Autodesk Fusion 360 part; units mm, degrees
note: some values were not read from the file. Chosen so that the rebuilt part matches the saved one: which bodies a step acts on; which face or edge a step refers to.
(part 2 of 3)
sketch "Sketch11 (2)" plane through (0, 171.45, 0) normal (0, 1, 0) x (-1, 0, 0) in component "enclosure"
  line L0 (75.40625, 30.353) -> (75.40625, -30.353)
  arc A0 (73.2155, -32.54375) -> (75.40625, -30.353) centre (73.2155, -30.353) ccw
  line L1 (73.2155, -32.54375) -> (-73.2155, -32.54375)
  arc A1 (-75.40625, -30.353) -> (-73.2155, -32.54375) centre (-73.2155, -30.353) ccw
  line L2 (-75.40625, -30.353) -> (-75.40625, 30.353)
  arc A2 (-73.2155, 32.54375) -> (-75.40625, 30.353) centre (-73.2155, 30.353) ccw
  line L3 (-73.2155, 32.54375) -> (73.2155, 32.54375)
  arc A3 (75.40625, 30.353) -> (73.2155, 32.54375) centre (73.2155, 30.353) ccw
  arc A4 (73.2155, -34.925) -> (77.7875, -30.353) centre (73.2155, -30.353) ccw
  line L4 (77.7875, -30.353) -> (77.7875, 30.353)
  arc A5 (77.7875, 30.353) -> (73.2155, 34.925) centre (73.2155, 30.353) ccw
  line L5 (73.2155, 34.925) -> (-73.2155, 34.925)
  arc A6 (-73.2155, 34.925) -> (-77.7875, 30.353) centre (-73.2155, 30.353) ccw
  line L6 (-77.7875, 30.353) -> (-77.7875, -30.353)
  arc A7 (-77.7875, -30.353) -> (-73.2155, -34.925) centre (-73.2155, -30.353) ccw
  line L7 (-73.2155, -34.925) -> (73.2155, -34.925)
  line L8 (-73.2155, 32.54375) -> (73.2155, 32.54375)
  line L9 (73.2155, 32.54375) -> (-73.2155, 32.54375)
  line L10 (73.2155, -32.54375) -> (-73.2155, -32.54375)
  line L11 (-73.2155, -32.54375) -> (73.2155, -32.54375)
  line L12 (-75.40625, -30.353) -> (-75.40625, 30.353)
  line L13 (-75.40625, 30.353) -> (-75.40625, -30.353)
  line L14 (75.40625, 30.353) -> (75.40625, -30.353)
  line L15 (75.40625, -30.353) -> (75.40625, 30.353)
  line L16 (0, 32.54375) -> (0, -32.54375) construction
  line L17 (-75.40625, 0) -> (0, 0) construction
  line L18 (-75.40625, 6.35) -> (-75.40625, -6.35)
  line L19 (-73.025, -3.96875) -> (-73.025, 3.96875)
  line L20 (-73.025, 6.35) -> (-75.40625, -6.35) construction
  line L21 (-75.40625, 6.35) -> (-73.025, -6.35) construction
  arc A8 (-73.025, 3.96875) -> (-75.40625, 6.35) centre (-75.40625, 3.96875) ccw
  arc A9 (-75.40625, -6.35) -> (-73.025, -3.96875) centre (-75.40625, -3.96875) ccw
  line L22 (73.025, -3.96875) -> (73.025, 3.96875)
  arc A10 (75.40625, 6.35) -> (73.025, 3.96875) centre (75.40625, 3.96875) ccw
  arc A11 (73.025, -3.96875) -> (75.40625, -6.35) centre (75.40625, -3.96875) ccw
  line L23 (75.40625, 6.35) -> (75.40625, -6.35)
  point P0 (-74.215625, 0)
  dimension "d154" = 12.7
  dimension "d155" = 2.38125
  dimension "d156" = 2.38125
  dimension "d157" = 2.38125
  constraint coincident L17.end origin
  constraint parallel L18 L19
  constraint coincident L20.start L19
  constraint tangent L19 A8
  constraint coincident L21.end L19
  constraint tangent L19 A9
  constraint collinear L2 L18
  constraint symmetric L16 A8 A10
  constraint symmetric L16 A9 A11
  measures "d156" radius of A8
  measures "d157" radius of A9
extrude "Extrude8'" add sketch "Sketch11 (2)" against normal up to surface (169.8625 mm away) contours L0 L14 L15 L22 A10 A11 L23 | L2 L12 L13 L18 L19 A8 A9 picked at (74.6125, -1.322917) picked at (-74.6125, -1.322917) bodies 2 in component "enclosure"
sketch "Sketch12" plane through (0, 171.45, 0) normal (0, 1, 0) x (-1, 0, 0) in component "enclosure"
  line L0 (75.40625, 30.353) -> (75.40625, 6.35)
  arc A0 (75.40625, 6.35) -> (73.025, 3.96875) centre (75.40625, 3.96875) ccw
  line L1 (73.025, 3.96875) -> (73.025, -3.96875)
  arc A1 (73.025, -3.96875) -> (75.40625, -6.35) centre (75.40625, -3.96875) ccw
  line L2 (75.40625, -6.35) -> (75.40625, -30.353)
  arc A2 (73.2155, -32.54375) -> (75.40625, -30.353) centre (73.2155, -30.353) ccw
  line L3 (73.2155, -32.54375) -> (-73.2155, -32.54375)
  arc A3 (-75.40625, -30.353) -> (-73.2155, -32.54375) centre (-73.2155, -30.353) ccw
  line L4 (-75.40625, -30.353) -> (-75.40625, -6.35)
  arc A4 (-75.40625, -6.35) -> (-73.025, -3.96875) centre (-75.40625, -3.96875) ccw
  line L5 (-73.025, -3.96875) -> (-73.025, 3.96875)
  arc A5 (-73.025, 3.96875) -> (-75.40625, 6.35) centre (-75.40625, 3.96875) ccw
  line L6 (-75.40625, 6.35) -> (-75.40625, 30.353)
  arc A6 (-73.2155, 32.54375) -> (-75.40625, 30.353) centre (-73.2155, 30.353) ccw
  line L7 (-73.2155, 32.54375) -> (73.2155, 32.54375)
  arc A7 (75.40625, 30.353) -> (73.2155, 32.54375) centre (73.2155, 30.353) ccw
  arc A8 (73.2155, -34.925) -> (77.7875, -30.353) centre (73.2155, -30.353) ccw
  line L8 (77.7875, -30.353) -> (77.7875, 30.353)
  arc A9 (77.7875, 30.353) -> (73.2155, 34.925) centre (73.2155, 30.353) ccw
  line L9 (73.2155, 34.925) -> (-73.2155, 34.925)
  arc A10 (-73.2155, 34.925) -> (-77.7875, 30.353) centre (-73.2155, 30.353) ccw
  line L10 (-77.7875, 30.353) -> (-77.7875, -30.353)
  arc A11 (-77.7875, -30.353) -> (-73.2155, -34.925) centre (-73.2155, -30.353) ccw
  line L11 (-73.2155, -34.925) -> (73.2155, -34.925)
  line L12 (-73.2155, 32.54375) -> (73.2155, 32.54375)
  line L13 (73.2155, 32.54375) -> (-73.2155, 32.54375)
  line L14 (73.2155, -32.54375) -> (-73.2155, -32.54375)
  line L15 (-73.2155, -32.54375) -> (73.2155, -32.54375)
  line L16 (-77.7875, 30.353) -> (-77.7875, -30.353)
  line L17 (-77.7875, -30.353) -> (-77.7875, 30.353)
  line L18 (77.7875, -30.353) -> (77.7875, 30.353)
  line L19 (77.7875, 30.353) -> (77.7875, -30.353)
  line L20 (-77.7875, 30.353) -> (-77.7875, -30.353) construction
  line L21 (-77.7875, 0) -> (0, 0) construction
  line L22 (-76.2, 0.79375) -> (-77.7875, 0.79375)
  line L23 (-77.7875, 0.79375) -> (-77.7875, -0.79375)
  line L24 (-77.7875, -0.79375) -> (-76.2, -0.79375)
  line L25 (-76.2, -0.79375) -> (-76.2, 0.79375)
  line L26 (-76.2, 0.79375) -> (-77.7875, -0.79375) construction
  line L27 (-77.7875, 0.79375) -> (-76.2, -0.79375) construction
  line L28 (0, 0) -> (0, -32.54375) construction
  line L29 (77.7875, 0.79375) -> (77.7875, -0.79375)
  line L30 (76.2, 0.79375) -> (77.7875, 0.79375)
  line L31 (76.2, -0.79375) -> (76.2, 0.79375)
  line L32 (77.7875, -0.79375) -> (76.2, -0.79375)
  point P0 (-76.99375, 0)
  dimension "d160" = 1.5875
  dimension "d161" = 1.5875
  constraint coincident A10.end L10.start
  constraint coincident L10.end A11.start
  constraint midpoint L16 L21.start
  constraint coincident L21.end L28.start
  constraint horizontal L22
  constraint perpendicular L22 L23
  constraint parallel L22 L24
  constraint parallel L23 L25
  constraint collinear L20 L23
extrude "Extrude9'" cut sketch "Sketch12" against normal up to surface (169.8625 mm away) contours L8 L18 L19 L29 L30 L31 L32 | L10 L16 L17 L22 L23 L24 L25 picked at (77.258333, -0.264583) picked at (-76.729167, -0.264583) bodies 2 in component "enclosure"
sketch "Sketch13" plane through (0, 171.45, 0) normal (0, 1, 0) x (-1, 0, 0) in component "enclosure"
  line L0 (-76.2, -0.79375) -> (-77.7875, -0.79375)
  line L1 (-77.7875, -0.79375) -> (-77.7875, -30.353)
  arc A0 (-77.7875, -30.353) -> (-73.2155, -34.925) centre (-73.2155, -30.353) ccw
  line L2 (-73.2155, -34.925) -> (73.2155, -34.925)
  arc A1 (73.2155, -34.925) -> (77.7875, -30.353) centre (73.2155, -30.353) ccw
  line L3 (77.7875, -30.353) -> (77.7875, -0.79375)
  line L4 (77.7875, -0.79375) -> (76.2, -0.79375)
  line L5 (76.2, -0.79375) -> (76.2, 0.79375)
  line L6 (76.2, 0.79375) -> (77.7875, 0.79375)
  line L7 (77.7875, 0.79375) -> (77.7875, 30.353)
  arc A2 (77.7875, 30.353) -> (73.2155, 34.925) centre (73.2155, 30.353) ccw
  line L8 (73.2155, 34.925) -> (-73.2155, 34.925)
  arc A3 (-73.2155, 34.925) -> (-77.7875, 30.353) centre (-73.2155, 30.353) ccw
  line L9 (-77.7875, 30.353) -> (-77.7875, 0.79375)
  line L10 (-77.7875, 0.79375) -> (-76.2, 0.79375)
  line L11 (-76.2, 0.79375) -> (-76.2, -0.79375)
  line L12 (75.40625, 30.353) -> (75.40625, 6.35)
  arc A4 (75.40625, 6.35) -> (73.025, 3.96875) centre (75.40625, 3.96875) ccw
  line L13 (73.025, 3.96875) -> (73.025, -3.96875)
  arc A5 (73.025, -3.96875) -> (75.40625, -6.35) centre (75.40625, -3.96875) ccw
  line L14 (75.40625, -6.35) -> (75.40625, -30.353)
  arc A6 (73.2155, -32.54375) -> (75.40625, -30.353) centre (73.2155, -30.353) ccw
  line L15 (73.2155, -32.54375) -> (-73.2155, -32.54375)
  arc A7 (-75.40625, -30.353) -> (-73.2155, -32.54375) centre (-73.2155, -30.353) ccw
  line L16 (-75.40625, -30.353) -> (-75.40625, -6.35)
  arc A8 (-75.40625, -6.35) -> (-73.025, -3.96875) centre (-75.40625, -3.96875) ccw
  line L17 (-73.025, -3.96875) -> (-73.025, 3.96875)
  arc A9 (-73.025, 3.96875) -> (-75.40625, 6.35) centre (-75.40625, 3.96875) ccw
  line L18 (-75.40625, 6.35) -> (-75.40625, 30.353)
  arc A10 (-73.2155, 32.54375) -> (-75.40625, 30.353) centre (-73.2155, 30.353) ccw
  line L19 (-73.2155, 32.54375) -> (73.2155, 32.54375)
  arc A11 (75.40625, 30.353) -> (73.2155, 32.54375) centre (73.2155, 30.353) ccw
  line L20 (-75.40625, 6.35) -> (-75.40625, 30.353) construction
  line L21 (-75.40625, 30.353) -> (-75.40625, 6.35) construction
  line L22 (75.40625, 6.35) -> (75.40625, 30.353) construction
  line L23 (75.40625, 30.353) -> (75.40625, 6.35) construction
  line L24 (-75.40625, -6.35) -> (-75.40625, -30.353) construction
  line L25 (-75.40625, -30.353) -> (-75.40625, -6.35) construction
  line L26 (75.40625, -6.35) -> (75.40625, -30.353) construction
  line L27 (75.40625, -30.353) -> (75.40625, -6.35) construction
  line L28 (-75.40625, 6.35) -> (75.40625, 6.35)
  line L29 (75.40625, 6.35) -> (75.40625, -6.35)
  line L30 (75.40625, -6.35) -> (-75.40625, -6.35)
  line L31 (-75.40625, -6.35) -> (-75.40625, 6.35)
  constraint horizontal L28
  constraint vertical L29
  constraint horizontal L30
  constraint vertical L31
extrude "Extrude10'" cut sketch "Sketch13" against normal blind 2.38125 contours A4 L13 A5 L29 | A8 L17 A9 L31 picked at (74.6125, -1.322917) picked at (-74.6125, -1.322917) bodies 2 in component "enclosure"
ref_plane "WorkPlane2" through (-74.215625, 169.06875, 0) normal (0, 1, 0) x (-1, 0, 0) in component "enclosure"
sketch "Sketch14 (2)" plane through (0, 169.06875, 0) normal (0, 1, 0) x (1, 0, 0) in component "enclosure"
  line L0 (73.2155, -32.54375) -> (-73.2155, -32.54375)
  line L1 (-73.2155, -32.54375) -> (73.2155, -32.54375)
  line L2 (-73.2155, 32.54375) -> (73.2155, 32.54375)
  line L3 (73.2155, 32.54375) -> (-73.2155, 32.54375)
  line L4 (75.40625, -6.35) -> (75.40625, -30.353)
  line L5 (75.40625, -30.353) -> (75.40625, 30.353)
  line L6 (75.40625, 30.353) -> (75.40625, 6.35)
  line L7 (75.40625, 6.35) -> (75.40625, -6.35)
  line L8 (-75.40625, 6.35) -> (-75.40625, 30.353)
  line L9 (-75.40625, 30.353) -> (-75.40625, -30.353)
  line L10 (-75.40625, -30.353) -> (-75.40625, -6.35)
  line L11 (-75.40625, -6.35) -> (-75.40625, 6.35)
  arc A0 (73.2155, -32.54375) -> (75.40625, -30.353) centre (73.2155, -30.353) ccw
  arc A1 (75.40625, 30.353) -> (73.2155, 32.54375) centre (73.2155, 30.353) ccw
  arc A2 (-75.40625, -30.353) -> (-73.2155, -32.54375) centre (-73.2155, -30.353) ccw
  arc A3 (-73.2155, 32.54375) -> (-75.40625, 30.353) centre (-73.2155, 30.353) ccw
  arc A4 (-73.2155, 32.54375) -> (-75.40625, 30.353) centre (-73.2155, 30.353) ccw
  arc A5 (-73.2155, 32.54375) -> (-75.40625, 30.353) centre (-73.2155, 30.353) ccw
  arc A6 (-75.40625, -30.353) -> (-73.2155, -32.54375) centre (-73.2155, -30.353) ccw
  arc A7 (-75.40625, -30.353) -> (-73.2155, -32.54375) centre (-73.2155, -30.353) ccw
  arc A8 (75.40625, 30.353) -> (73.2155, 32.54375) centre (73.2155, 30.353) ccw
  arc A9 (75.40625, 30.353) -> (73.2155, 32.54375) centre (73.2155, 30.353) ccw
  arc A10 (73.2155, -32.54375) -> (75.40625, -30.353) centre (73.2155, -30.353) ccw
  arc A11 (73.2155, -32.54375) -> (75.40625, -30.353) centre (73.2155, -30.353) ccw
  line L12 (0, 0) -> (0, -32.54375) construction
  line L13 (0, 0) -> (75.40625, 0) construction
  line L14 (73.2155, -32.54375) -> (92.352054, -32.54375) construction
  line L15 (75.40625, -30.353) -> (75.40625, -49.403) construction
  line L16 (75.40625, -32.54375) -> (62.70625, -32.54375)
  line L17 (62.70625, -32.54375) -> (62.70625, -19.84375)
  line L18 (62.70625, -19.84375) -> (75.40625, -19.84375)
  line L19 (75.40625, -19.84375) -> (75.40625, -32.54375)
  line L20 (75.40625, -19.84375) -> (62.70625, -32.54375) construction
  line L21 (62.70625, -19.84375) -> (75.40625, -32.54375) construction
  circle A12 centre (69.05625, -26.19375) radius 1.785937
  circle A13 centre (-69.05625, -26.19375) radius 1.785937
  line L22 (-62.70625, -32.54375) -> (-62.70625, -19.84375)
  line L23 (-62.70625, -19.84375) -> (-75.40625, -19.84375)
  line L24 (62.70625, 19.84375) -> (75.40625, 19.84375)
  line L25 (62.70625, 32.54375) -> (62.70625, 19.84375)
  circle A14 centre (69.05625, 26.19375) radius 1.785937
  circle A15 centre (-69.05625, 26.19375) radius 1.785937
  line L26 (-62.70625, 19.84375) -> (-75.40625, 19.84375)
  line L27 (-62.70625, 32.54375) -> (-62.70625, 19.84375)
  point P0 (75.40625, -32.54375)
  point P1 (69.05625, -26.19375)
  dimension "d167" = 19.05
  dimension "d172" = 12.7
  dimension "d173" = 12.7
  dimension "d174" = 3.571875
  constraint coincident L12.start L13.start
  constraint tangent A11 L14
  constraint parallel L1 L14
  constraint parallel L5 L15
  constraint horizontal L16
  constraint vertical L17
  constraint horizontal L18
  constraint vertical L19
  constraint symmetric L12 A12 A13
  constraint symmetric L13 A12 A14
  constraint symmetric L13 A13 A15
  measures "d174" diameter of A12
extrude "Extrude11" add sketch "Sketch14 (2)" against normal blind 12.7 contours L0 L1 L4 L5 A0 A10 A11 L16 L17 L18 L19 | L0 L1 L9 L10 A2 A6 A7 L22 L23 | L2 L3 L5 L6 A1 A8 A9 L24 L25 | L2 L3 L8 L9 A3 A4 A5 L26 L27 picked at (69.100738, -21.366769) picked at (-69.011762, -21.366769) picked at (69.011762, 21.366769) picked at (-69.011762, 21.366769) bodies 2 in component "enclosure"
sketch "Sketch15 (2)" plane through (0, 156.36875, 0) normal (0, -1, 0) x (1, 0, 0) in component "enclosure"
  circle A0 centre (-69.05625, 26.19375) radius 1.785938
  arc A1 (-73.2155, 32.54375) -> (-75.40625, 30.353) centre (-73.2155, 30.353) ccw
  line L0 (-75.40625, 30.353) -> (-75.40625, 19.84375)
  line L1 (-75.40625, 19.84375) -> (-62.70625, 19.84375)
  line L2 (-62.70625, 19.84375) -> (-62.70625, 32.54375)
  line L3 (-62.70625, 32.54375) -> (-73.2155, 32.54375)
  circle A2 centre (-69.05625, 26.19375) radius 2.69875
  line L4 (0, 0) -> (0, 30.480001) construction
  line L5 (0, 0) -> (-67.323683, 0) construction
  circle A3 centre (69.05625, 26.19375) radius 2.69875
  circle A4 centre (69.05625, -26.19375) radius 2.69875
  circle A5 centre (-69.05625, -26.19375) radius 2.69875
  circle A6 centre (-69.05625, 26.19375) radius 1.785937
  circle A7 centre (69.05625, 26.19375) radius 1.785937
  circle A8 centre (-69.05625, -26.19375) radius 1.785937
  circle A9 centre (69.05625, -26.19375) radius 1.785937
  dimension "d177" = 3.571875
  constraint concentric A0 A2
  constraint coincident L4.start L5.start
  constraint vertical L4
  constraint perpendicular L4 L5
  constraint symmetric A2 L4 A3
  constraint symmetric A2 L5 A5
  constraint symmetric L5 A3 A4
  constraint concentric A2 A6
  constraint symmetric L4 A6 A7
  constraint symmetric L5 A6 A8
  constraint symmetric L5 A7 A9
  measures "d177" diameter of A6
extrude "Extrude12'" add sketch "Sketch15 (2)" against normal up to surface (3.175 mm away) contours A2 | A3 | A4 | A5 picked at (-70.438094, 28.141569) picked at (67.674406, 28.141569) picked at (67.674406, -24.245931) picked at (-70.438094, -24.245931) bodies 2 in component "enclosure"
sketch "Sketch18" plane through (0, -19.05, 0) normal (0, -1, 0) x (1, 0, 0) in component "face"
  line L0 (52.6415, -5.535649) -> (-52.6415, -5.535649)
  line L1 (-52.6415, -5.535649) -> (-52.6415, 22.642476)
  line L2 (-52.6415, 22.642476) -> (52.6415, 22.642476)
  line L3 (52.6415, 22.642476) -> (52.6415, -5.535649)
  line L4 (71.4375, -15.145606) -> (71.4375, -17.526856)
  line L5 (71.4375, -17.526856) -> (-71.4375, -17.526856)
  line L6 (-71.4375, -17.526856) -> (-71.4375, -15.145606)
  line L7 (-71.4375, -15.145606) -> (71.4375, -15.145606)
  ellipse E0 centre (-72.882285, -30.019785) end of major axis (-76.116162, -33.253662) minor radius 4.572 (-77.454981, -30.021177) -> (-72.883677, -34.592481) ccw
  line L8 (-72.883677, -34.592481) -> (72.883677, -34.592481)
  ellipse E1 centre (72.882285, -30.019785) end of major axis (76.116162, -33.253662) minor radius 4.572 (72.883677, -34.592481) -> (77.454981, -30.021177) ccw
  line L9 (77.454981, -30.021177) -> (77.454981, 30.021177)
  ellipse E2 centre (72.882285, 30.019785) end of major axis (76.116162, 33.253662) minor radius 4.572 (77.454981, 30.021177) -> (72.883677, 34.592481) ccw
  line L10 (72.883677, 34.592481) -> (-72.883677, 34.592481)
  ellipse E3 centre (-72.882285, 30.019785) end of major axis (-76.116162, 33.253662) minor radius 4.572 (-72.883677, 34.592481) -> (-77.454981, 30.021177) ccw
  line L11 (-77.454981, 30.021177) -> (-77.454981, -30.021177)
  line L12 (-71.104981, 28.242481) -> (-58.404981, 28.242481)
  line L13 (-58.404981, 28.242481) -> (-58.404981, 15.542481)
  line L14 (-58.404981, 15.542481) -> (-71.104981, 15.542481)
  line L15 (-71.104981, 15.542481) -> (-71.104981, 28.242481)
  line L16 (-64.754981, 28.242481) -> (-64.754981, 34.592481) construction
  line L17 (-71.104981, 21.892481) -> (-77.454981, 21.892481) construction
  dimension "d182" = 12.7
  dimension "d183" = 12.7
  dimension "d184" = 6.35
  dimension "d185" = 6.35
  constraint horizontal L12
  constraint vertical L13
  constraint horizontal L14
  constraint vertical L15
  constraint perpendicular L10 L16
  constraint perpendicular L11 L17
extrude "Extrude13" cut sketch "Sketch18" against normal blind 1.5875 contours L12 L13 L14 L15 picked at (-66.871648, 19.775814) bodies 1 in component "face"
sketch "Sketch19" plane through (0, -16.66875, 0) normal (0, 1, 0) x (-1, 0, 0) in component "face"
  line L0 (-50.26025, 20.261226) -> (50.26025, 20.261226)
  line L1 (50.26025, 20.261226) -> (50.26025, -3.154399)
  line L2 (50.26025, -3.154399) -> (-50.26025, -3.154399)
  line L3 (-50.26025, -3.154399) -> (-50.26025, 20.261226)
  line L4 (-53.43525, -3.948149) -> (53.43525, -3.948149)
  line L5 (53.43525, -3.948149) -> (53.43525, -6.329399)
  line L6 (53.43525, -6.329399) -> (-53.43525, -6.329399)
  line L7 (-53.43525, -6.329399) -> (-53.43525, -3.948149)
  ellipse E0 centre (72.923849, -30.061349) end of major axis (74.473416, -31.610916) minor radius 2.19075 (72.924517, -32.252433) -> (75.114933, -30.062017) ccw
  line L8 (75.114933, -30.062017) -> (75.114933, 30.062017)
  ellipse E1 centre (72.923849, 30.061349) end of major axis (74.473416, 31.610916) minor radius 2.19075 (75.114933, 30.062017) -> (72.924517, 32.252433) ccw
  line L9 (72.924517, 32.252433) -> (-72.924517, 32.252433)
  ellipse E2 centre (-72.923849, 30.061349) end of major axis (-74.473416, 31.610916) minor radius 2.19075 (-72.924517, 32.252433) -> (-75.114933, 30.062017) ccw
  line L10 (-75.114933, 30.062017) -> (-75.114933, -30.062017)
  ellipse E3 centre (-72.923849, -30.061349) end of major axis (-74.473416, -31.610916) minor radius 2.19075 (-75.114933, -30.062017) -> (-72.924517, -32.252433) ccw
  line L11 (-72.924517, -32.252433) -> (72.924517, -32.252433)
  line L12 (-71.4375, -17.526856) -> (-71.4375, -15.145606)
  line L13 (-71.4375, -15.145606) -> (71.4375, -15.145606)
  line L14 (71.4375, -15.145606) -> (71.4375, -17.526856)
  line L15 (71.4375, -17.526856) -> (-71.4375, -17.526856)
  line L16 (53.43525, 21.054976) -> (-53.43525, 21.054976)
  line L17 (-53.43525, 21.054976) -> (-53.43525, 23.436226)
  line L18 (-53.43525, 23.436226) -> (53.43525, 23.436226)
  line L19 (53.43525, 23.436226) -> (53.43525, 21.054976)
  line L20 (71.104981, 15.542481) -> (71.104981, 28.242481)
  line L21 (71.104981, 28.242481) -> (58.404981, 28.242481)
  line L22 (71.104981, 28.242481) -> (58.404981, 28.242481)
  line L23 (58.404981, 28.242481) -> (58.404981, 15.542481)
  line L24 (58.404981, 15.542481) -> (71.104981, 15.542481)
  line L25 (71.104981, 15.542481) -> (71.104981, 28.242481)
  dimension "d189" = 12.7
  dimension "d190" = 12.7
  constraint horizontal L22
  constraint vertical L23
  constraint horizontal L24
  constraint vertical L25
extrude "Extrude14" add sketch "Sketch19" along normal blind 1.5875 contours L20 L21 L22 L23 L24 L25 picked at (62.638314, 19.775814) bodies 1 in component "face"
chamfer "Chamfer1'" distance 1.5875 angle 45 4 edges at (-64.754981, -16.66875, 15.542481) (-71.104981, -16.66875, 21.892481) (-64.754981, -16.66875, 28.242481) (-58.404981, -16.66875, 21.892481) on bodies 1 in component "face"
ref_plane "WorkPlane1" through (-64.754981, -17.4625, 21.892481) normal (0, -1, 0) x (0, 0, -1) in component "badge"
sketch "Sketch1 (2)" plane through (0, -17.4625, 0) normal (0, -1, 0) x (-1, 0, 0) in component "badge"
  line L0 (58.404981, -28.242481) -> (71.104981, -28.242481)
  line L1 (71.104981, -28.242481) -> (58.404981, -28.242481)
  line L2 (71.104981, -28.242481) -> (71.104981, -15.542481)
  line L3 (71.104981, -15.542481) -> (71.104981, -28.242481)
  line L4 (71.104981, -28.242481) -> (58.404981, -28.242481)
  line L5 (58.404981, -28.242481) -> (58.404981, -15.542481)
  line L6 (58.404981, -15.542481) -> (71.104981, -15.542481)
  line L7 (71.104981, -15.542481) -> (71.104981, -28.242481)
  dimension "d195" = 12.7
  dimension "d196" = 12.7
  constraint horizontal L4
  constraint vertical L5
  constraint horizontal L6
  constraint vertical L7
extrude "Extrude1''" add sketch "Sketch1 (2)" along normal blind 1.5875 separate body makes body 8 in component "badge"
sketch "Sketch2 (3)" plane through (0, -19.05, 0) normal (0, -1, 0) x (1, 0, 0) in component "badge"
  line L0 (-71.104981, 15.542481) -> (-58.404981, 15.542481)
  line L1 (-58.404981, 15.542481) -> (-58.404981, 28.242481)
  line L2 (-58.404981, 28.242481) -> (-71.104981, 28.242481)
  line L3 (-71.104981, 28.242481) -> (-71.104981, 15.542481)
sketch "Sketch3 (2)" plane through (0, -19.05, 0) normal (0, -1, 0) x (1, 0, 0) in component "badge"
  line L0 (-68.609781, 21.776665) -> (-67.4942, 21.776665)
  line L1 (-66.849908, 17.9646) -> (-65.873463, 17.9646)
  line L2 (-59.360374, 25.729423) -> (-65.873463, 17.9646)
  line L3 (-59.360374, 25.729423) -> (-60.451999, 25.729423)
  line L4 (-60.451999, 25.729423) -> (-66.168356, 18.914454)
  line L5 (-68.609781, 21.776665) -> (-67.4942, 21.776665)
  line L6 (-60.451999, 25.729423) -> (-66.168356, 18.914454)
  line L7 (-59.360374, 25.729423) -> (-60.451999, 25.729423)
  line L8 (-59.360374, 25.729423) -> (-65.873463, 17.9646)
  line L9 (-66.849908, 17.9646) -> (-65.873463, 17.9646)
  line L10 (-68.609781, 21.776665) -> (-67.4942, 21.776665)
  line L11 (-60.451999, 25.729423) -> (-66.168356, 18.914454)
  line L12 (-59.360374, 25.729423) -> (-65.873463, 17.9646)
  line L13 (-66.849908, 17.9646) -> (-65.873463, 17.9646)
  line L14 (-59.360374, 25.729423) -> (-60.451999, 25.729423)
  line L15 (-70.147672, 21.776665) -> (-69.032091, 21.776665)
  line L16 (-70.147672, 21.776665) -> (-68.387798, 17.9646)
  line L17 (-69.032091, 21.776665) -> (-67.706247, 18.914454)
  line L18 (-68.387798, 17.9646) -> (-67.411354, 17.9646)
  line L19 (-60.898265, 25.729423) -> (-61.98989, 25.729423)
  line L20 (-68.609781, 21.776665) -> (-67.436746, 19.23575)
  line L21 (-67.04922, 18.396331) -> (-66.849908, 17.9646)
  line L22 (-61.98989, 25.729423) -> (-66.715497, 20.095613)
  line L23 (-67.436746, 19.23575) -> (-67.706247, 18.914454)
  line L24 (-68.609781, 21.776665) -> (-67.436746, 19.23575)
  line L25 (-67.04922, 18.396331) -> (-66.849908, 17.9646)
  line L26 (-68.609781, 21.776665) -> (-67.436746, 19.23575)
  line L27 (-67.04922, 18.396331) -> (-66.849908, 17.9646)
  line L28 (-67.4942, 21.776665) -> (-66.715497, 20.095613)
  line L29 (-66.327126, 19.257203) -> (-66.168356, 18.914454)
  line L30 (-67.4942, 21.776665) -> (-66.715497, 20.095613)
  line L31 (-66.327126, 19.257203) -> (-66.168356, 18.914454)
  line L32 (-67.4942, 21.776665) -> (-66.715497, 20.095613)
  line L33 (-66.327126, 19.257203) -> (-66.168356, 18.914454)
  line L34 (-60.898265, 25.729423) -> (-66.327126, 19.257203)
  line L35 (-67.04922, 18.396331) -> (-67.411354, 17.9646)
  constraint horizontal L0
  constraint horizontal L1
  constraint horizontal L3
  constraint parallel L2 L4
  constraint horizontal L5
  constraint horizontal L9
  constraint horizontal L7
  constraint parallel L6 L8
  constraint horizontal L10
  constraint horizontal L13
  constraint horizontal L14
  constraint horizontal L19
  constraint horizontal L15
  constraint horizontal L18
  constraint collinear L20 L21
  constraint collinear L22 L23
  constraint collinear L24 L25
  constraint collinear L26 L27
  constraint collinear L28 L29
  constraint collinear L30 L31
  constraint collinear L32 L33
  constraint collinear L34 L35
extrude "Extrude2'" add sketch "Sketch3 (2)" along normal blind 0.396875 bodies 8 in component "badge"
sketch "Sketch16 (2)" plane through (0, 0, -34.925) normal (0, 0, -1) x (1, 0, 0) in component "enclosure"
  line L0 (73.2155, -1.5875) -> (-73.2155, -1.5875)
  line L1 (-73.2155, -1.5875) -> (-73.2155, -171.45)
  line L2 (-73.2155, -171.45) -> (73.2155, -171.45)
  line L3 (73.2155, -171.45) -> (73.2155, -1.5875)
  line L4 (-77.7875, -1.5875) -> (-77.7875, -171.45)
  line L5 (-77.7875, -171.45) -> (-77.7875, -1.5875)
  line L6 (77.7875, -171.45) -> (77.7875, -1.5875)
  line L7 (77.7875, -1.5875) -> (77.7875, -171.45)
  line L8 (-77.7875, -1.5875) -> (77.7875, -1.5875) construction
  line L9 (-77.7875, -171.45) -> (77.7875, -171.45) construction
  line L10 (0, -171.45) -> (0, -1.5875) construction
  line L11 (-58.7375, -7.9375) -> (-39.6875, -7.9375)
  line L12 (-39.6875, -7.9375) -> (-39.6875, -26.9875)
  line L13 (-39.6875, -26.9875) -> (-58.7375, -26.9875)
  line L14 (-58.7375, -26.9875) -> (-58.7375, -7.9375)
  line L15 (-58.7375, -17.4625) -> (-77.7875, -17.4625) construction
  line L16 (-49.2125, -7.9375) -> (-49.2125, -1.5875) construction
  line L17 (-58.7375, -152.4) -> (-39.6875, -152.4)
  line L18 (-39.6875, -152.4) -> (-39.6875, -133.35)
  line L19 (-39.6875, -133.35) -> (-58.7375, -133.35)
  line L20 (-58.7375, -133.35) -> (-58.7375, -152.4)
  line L21 (-58.7375, -142.875) -> (-77.7875, -142.875) construction
  line L22 (-49.2125, -152.4) -> (-49.2125, -171.45) construction
  line L23 (39.6875, -152.4) -> (39.6875, -133.35)
  line L24 (39.6875, -133.35) -> (58.7375, -133.35)
  line L25 (58.7375, -152.4) -> (39.6875, -152.4)
  line L26 (39.6875, -7.9375) -> (39.6875, -26.9875)
  line L27 (39.6875, -26.9875) -> (58.7375, -26.9875)
  line L28 (58.7375, -7.9375) -> (39.6875, -7.9375)
  line L29 (58.7375, -26.9875) -> (58.7375, -7.9375)
  line L30 (58.7375, -133.35) -> (58.7375, -152.4)
  dimension "d205" = 19.05
  dimension "d206" = 19.05
  dimension "d207" = 19.05
  dimension "d208" = 6.35
  dimension "d209" = 19.05
  dimension "d210" = 19.05
  dimension "d211" = 19.05
  dimension "d212" = 19.05
  constraint coincident L4.start L5.end
  constraint coincident L6.end L7.start
  constraint coincident L4.end L5.start
  constraint coincident L6.start L7.end
  constraint midpoint L9 L10.start
  constraint midpoint L0 L10.end
  constraint horizontal L11
  constraint vertical L12
  constraint horizontal L13
  constraint vertical L14
  constraint midpoint L14 L15.start
  constraint coincident L4 L15.end
  constraint perpendicular L4 L15
  constraint vertical L16
  constraint midpoint L11 L16.start
  constraint coincident L8 L16.end
  constraint horizontal L17
  constraint vertical L18
  constraint horizontal L19
  constraint vertical L20
  constraint midpoint L20 L21.start
  constraint coincident L4 L21.end
  constraint perpendicular L4 L21
  constraint vertical L22
  constraint midpoint L17 L22.start
  constraint coincident L9 L22.end
  constraint symmetric L10 L11.start L28.start
  constraint symmetric L10 L11.end L26.start
  constraint symmetric L10 L12.end L26.end
  constraint symmetric L10 L13.end L27.end
  constraint symmetric L10 L17.start L25.start
  constraint symmetric L10 L17.end L23.start
  constraint symmetric L10 L18.end L23.end
  constraint symmetric L10 L19.end L24.end
  measures "d205" distance of L11.start L11.end
  measures "d206" distance of L11.start L13.end
  measures "d207" distance of L15.start L15.end
  measures "d208" distance of L16.start L16.end
  measures "d209" distance of L17.start L17.end
  measures "d210" distance of L17.start L19.end
  measures "d211" distance of L21.start L21.end
  measures "d212" distance of L22.start L22.end
extrude "Extrude13'" cut sketch "Sketch16 (2)" against normal blind 0.79375 contours L11 L12 L13 L14 | L17 L18 L19 L20 | L23 L24 L25 L30 | L26 L27 L28 L29 picked at (-52.3875, -14.2875) picked at (-52.3875, -139.7) picked at (46.0375, -139.7) picked at (46.0375, -14.2875) bodies 2 in component "enclosure"
sketch "Sketch18 (2)" plane through (0, 0, -34.925) normal (0, 0, -1) x (1, 0, 0) in component "enclosure"
  line L0 (-39.6875, -7.9375) -> (-39.6875, -26.9875)
  line L1 (-39.6875, -26.9875) -> (-58.7375, -26.9875)
  line L2 (-58.7375, -26.9875) -> (-58.7375, -7.9375)
  line L3 (-58.7375, -7.9375) -> (-39.6875, -7.9375)
  line L4 (-39.6875, -152.4) -> (-58.7375, -152.4)
  line L5 (-58.7375, -152.4) -> (-58.7375, -133.35)
  line L6 (-58.7375, -133.35) -> (-39.6875, -133.35)
  line L7 (-39.6875, -133.35) -> (-39.6875, -152.4)
  line L8 (39.6875, -7.9375) -> (58.7375, -7.9375)
  line L9 (58.7375, -7.9375) -> (58.7375, -26.9875)
  line L10 (58.7375, -26.9875) -> (39.6875, -26.9875)
  line L11 (39.6875, -26.9875) -> (39.6875, -7.9375)
  line L12 (39.6875, -152.4) -> (39.6875, -133.35)
  line L13 (39.6875, -133.35) -> (58.7375, -133.35)
  line L14 (58.7375, -133.35) -> (58.7375, -152.4)
  line L15 (58.7375, -152.4) -> (39.6875, -152.4)
  line L16 (73.2155, -1.5875) -> (-73.2155, -1.5875)
  line L17 (-73.2155, -1.5875) -> (-73.2155, -171.45)
  line L18 (-73.2155, -171.45) -> (73.2155, -171.45)
  line L19 (73.2155, -171.45) -> (73.2155, -1.5875)
  line L20 (-39.6875, -17.4625) -> (39.6875, -17.4625) construction
  line L21 (-0.79375, -23.8125) -> (0.79375, -23.8125)
  line L22 (0.79375, -23.8125) -> (0.79375, -11.1125)
  line L23 (0.79375, -11.1125) -> (-0.79375, -11.1125)
  line L24 (-0.79375, -11.1125) -> (-0.79375, -23.8125)
  line L25 (-0.79375, -23.8125) -> (0.79375, -11.1125) construction
  line L26 (0.79375, -23.8125) -> (-0.79375, -11.1125) construction
  line L27 (-36.115625, -11.1125) -> (-37.703125, -11.1125)
  line L28 (-36.115625, -23.8125) -> (-36.115625, -11.1125)
  line L29 (-37.703125, -23.8125) -> (-36.115625, -23.8125)
  line L30 (-37.703125, -11.1125) -> (-37.703125, -23.8125)
  line L31 (-28.73375, -11.1125) -> (-30.32125, -11.1125)
  line L32 (-28.73375, -23.8125) -> (-28.73375, -11.1125)
  line L33 (-30.32125, -23.8125) -> (-28.73375, -23.8125)
  line L34 (-30.32125, -11.1125) -> (-30.32125, -23.8125)
  line L35 (-21.351875, -11.1125) -> (-22.939375, -11.1125)
  line L36 (-21.351875, -23.8125) -> (-21.351875, -11.1125)
  line L37 (-22.939375, -23.8125) -> (-21.351875, -23.8125)
  line L38 (-22.939375, -11.1125) -> (-22.939375, -23.8125)
  line L39 (-13.97, -11.1125) -> (-15.5575, -11.1125)
  line L40 (-13.97, -23.8125) -> (-13.97, -11.1125)
  line L41 (-15.5575, -23.8125) -> (-13.97, -23.8125)
  line L42 (-15.5575, -11.1125) -> (-15.5575, -23.8125)
  line L43 (-6.588125, -11.1125) -> (-8.175625, -11.1125)
  line L44 (-6.588125, -23.8125) -> (-6.588125, -11.1125)
  line L45 (-8.175625, -23.8125) -> (-6.588125, -23.8125)
  line L46 (-8.175625, -11.1125) -> (-8.175625, -23.8125)
  line L47 (8.175625, -11.1125) -> (6.588125, -11.1125)
  line L48 (8.175625, -23.8125) -> (8.175625, -11.1125)
  line L49 (6.588125, -23.8125) -> (8.175625, -23.8125)
  line L50 (6.588125, -11.1125) -> (6.588125, -23.8125)
  line L51 (15.5575, -11.1125) -> (13.97, -11.1125)
  line L52 (15.5575, -23.8125) -> (15.5575, -11.1125)
  line L53 (13.97, -23.8125) -> (15.5575, -23.8125)
  line L54 (13.97, -11.1125) -> (13.97, -23.8125)
  line L55 (22.939375, -11.1125) -> (21.351875, -11.1125)
  line L56 (22.939375, -23.8125) -> (22.939375, -11.1125)
  line L57 (21.351875, -23.8125) -> (22.939375, -23.8125)
  line L58 (21.351875, -11.1125) -> (21.351875, -23.8125)
  line L59 (30.32125, -11.1125) -> (28.73375, -11.1125)
  line L60 (30.32125, -23.8125) -> (30.32125, -11.1125)
  line L61 (28.73375, -23.8125) -> (30.32125, -23.8125)
  line L62 (28.73375, -11.1125) -> (28.73375, -23.8125)
  line L63 (37.703125, -11.1125) -> (36.115625, -11.1125)
  line L64 (37.703125, -23.8125) -> (37.703125, -11.1125)
  line L65 (36.115625, -23.8125) -> (37.703125, -23.8125)
  line L66 (36.115625, -11.1125) -> (36.115625, -23.8125)
  point P0 (0, -17.4625)
  dimension "d223" = 1.5875
  dimension "d224" = 12.7
  dimension "d227" = 36.909375
  dimension "d228" = 0
  constraint midpoint L0 L20.start
  constraint midpoint L11 L20.end
  constraint horizontal L21
  constraint perpendicular L21 L22
  constraint parallel L21 L23
  constraint parallel L22 L24
  constraint coincident L25 P0
  constraint coincident L26 P0
  constraint midpoint L20 P0
extrude "Extrude14'" cut sketch "Sketch18 (2)" against normal up to surface (6.35 mm away) contours L21 L22 L23 L24 | L27 L28 L29 L30 | L31 L32 L33 L34 | L35 L36 L37 L38 | L39 L40 L41 L42 | L43 L44 L45 L46 | L47 L48 L49 L50 | L51 L52 L53 L54 | L55 L56 L57 L58 | L59 L60 L61 L62 | L63 L64 L65 L66 picked at (-0.264583, -15.345833) picked at (-37.173958, -15.345833) picked at (-29.262917, -19.579167) picked at (-22.410208, -15.345833) picked at (-15.028333, -15.345833) picked at (-7.646458, -15.345833) picked at (7.117292, -15.345833) picked at (14.499167, -15.345833) picked at (21.881042, -15.345833) picked at (29.792083, -19.579167) picked at (36.644792, -15.345833) bodies 2 in component "enclosure"
sketch "Sketch19 (2)" plane through (0, 0, -34.925) normal (0, 0, -1) x (1, 0, 0) in component "enclosure"
  line L0 (21.351875, -11.1125) -> (22.939375, -11.1125)
  line L1 (22.939375, -11.1125) -> (22.939375, -23.8125)
  line L2 (22.939375, -23.8125) -> (21.351875, -23.8125)
  line L3 (21.351875, -23.8125) -> (21.351875, -11.1125)
  line L4 (-30.32125, -11.1125) -> (-28.73375, -11.1125)
  line L5 (-28.73375, -11.1125) -> (-28.73375, -23.8125)
  line L6 (-28.73375, -23.8125) -> (-30.32125, -23.8125)
  line L7 (-30.32125, -23.8125) -> (-30.32125, -11.1125)
  line L8 (-0.79375, -11.1125) -> (0.79375, -11.1125)
  line L9 (0.79375, -11.1125) -> (0.79375, -23.8125)
  line L10 (0.79375, -23.8125) -> (-0.79375, -23.8125)
  line L11 (-0.79375, -23.8125) -> (-0.79375, -11.1125)
  line L12 (-22.939375, -11.1125) -> (-21.351875, -11.1125)
  line L13 (-21.351875, -11.1125) -> (-21.351875, -23.8125)
  line L14 (-21.351875, -23.8125) -> (-22.939375, -23.8125)
  line L15 (-22.939375, -23.8125) -> (-22.939375, -11.1125)
  line L16 (13.97, -11.1125) -> (15.5575, -11.1125)
  line L17 (15.5575, -11.1125) -> (15.5575, -23.8125)
  line L18 (15.5575, -23.8125) -> (13.97, -23.8125)
  line L19 (13.97, -23.8125) -> (13.97, -11.1125)
  line L20 (28.73375, -11.1125) -> (30.32125, -11.1125)
  line L21 (30.32125, -11.1125) -> (30.32125, -23.8125)
  line L22 (30.32125, -23.8125) -> (28.73375, -23.8125)
  line L23 (28.73375, -23.8125) -> (28.73375, -11.1125)
  line L24 (-37.703125, -11.1125) -> (-36.115625, -11.1125)
  line L25 (-36.115625, -11.1125) -> (-36.115625, -23.8125)
  line L26 (-36.115625, -23.8125) -> (-37.703125, -23.8125)
  line L27 (-37.703125, -23.8125) -> (-37.703125, -11.1125)
  line L28 (-8.175625, -11.1125) -> (-6.588125, -11.1125)
  line L29 (-6.588125, -11.1125) -> (-6.588125, -23.8125)
  line L30 (-6.588125, -23.8125) -> (-8.175625, -23.8125)
  line L31 (-8.175625, -23.8125) -> (-8.175625, -11.1125)
  line L32 (-15.5575, -11.1125) -> (-13.97, -11.1125)
  line L33 (-13.97, -11.1125) -> (-13.97, -23.8125)
  line L34 (-13.97, -23.8125) -> (-15.5575, -23.8125)
  line L35 (-15.5575, -23.8125) -> (-15.5575, -11.1125)
  line L36 (6.588125, -11.1125) -> (8.175625, -11.1125)
  line L37 (8.175625, -11.1125) -> (8.175625, -23.8125)
  line L38 (8.175625, -23.8125) -> (6.588125, -23.8125)
  line L39 (6.588125, -23.8125) -> (6.588125, -11.1125)
  line L40 (36.115625, -11.1125) -> (37.703125, -11.1125)
  line L41 (37.703125, -11.1125) -> (37.703125, -23.8125)
  line L42 (37.703125, -23.8125) -> (36.115625, -23.8125)
  line L43 (36.115625, -23.8125) -> (36.115625, -11.1125)
  line L44 (-39.6875, -7.9375) -> (-39.6875, -26.9875)
  line L45 (-39.6875, -26.9875) -> (-58.7375, -26.9875)
  line L46 (-58.7375, -26.9875) -> (-58.7375, -7.9375)
  line L47 (-58.7375, -7.9375) -> (-39.6875, -7.9375)
  line L48 (-39.6875, -152.4) -> (-58.7375, -152.4)
  line L49 (-58.7375, -152.4) -> (-58.7375, -133.35)
  line L50 (-58.7375, -133.35) -> (-39.6875, -133.35)
  line L51 (-39.6875, -133.35) -> (-39.6875, -152.4)
  line L52 (39.6875, -7.9375) -> (58.7375, -7.9375)
  line L53 (58.7375, -7.9375) -> (58.7375, -26.9875)
  line L54 (58.7375, -26.9875) -> (39.6875, -26.9875)
  line L55 (39.6875, -26.9875) -> (39.6875, -7.9375)
  line L56 (39.6875, -152.4) -> (39.6875, -133.35)
  line L57 (39.6875, -133.35) -> (58.7375, -133.35)
  line L58 (58.7375, -133.35) -> (58.7375, -152.4)
  line L59 (58.7375, -152.4) -> (39.6875, -152.4)
  line L60 (73.2155, -1.5875) -> (-73.2155, -1.5875)
  line L61 (-73.2155, -1.5875) -> (-73.2155, -171.45)
  line L62 (-73.2155, -171.45) -> (73.2155, -171.45)
  line L63 (73.2155, -171.45) -> (73.2155, -1.5875)
  line L64 (-73.2155, -1.5875) -> (73.2155, -171.45) construction
  line L65 (-25.4, -124.61875) -> (25.4, -124.61875)
  line L66 (25.4, -124.61875) -> (25.4, -48.41875)
  line L67 (25.4, -48.41875) -> (-25.4, -48.41875)
  line L68 (-25.4, -48.41875) -> (-25.4, -124.61875)
  line L69 (-25.4, -124.61875) -> (25.4, -48.41875) construction
  line L70 (25.4, -124.61875) -> (-25.4, -48.41875) construction
  point P0 (0, -86.51875)
  dimension "d233" = 50.8
  dimension "d234" = 76.2
  constraint coincident L60.end L61.start
  constraint coincident L62.end L63.start
  constraint horizontal L65
  constraint perpendicular L65 L66
  constraint parallel L65 L67
  constraint parallel L66 L68
extrude "Extrude15" cut sketch "Sketch19 (2)" against normal blind 0.79375 contours L65 L66 L67 L68 picked at (8.466667, -73.81875) bodies 2 in component "enclosure"
sketch "Sketch21" plane through (0, 0, 34.925) normal (0, 0, 1) x (-1, 0, 0) in component "enclosure"
  line L0 (73.2155, -1.5875) -> (-73.2155, -1.5875)
  line L1 (-73.2155, -1.5875) -> (-73.2155, -171.45)
  line L2 (-73.2155, -171.45) -> (73.2155, -171.45)
  line L3 (73.2155, -171.45) -> (73.2155, -1.5875)
  line L4 (77.7875, -171.45) -> (77.7875, -1.5875)
  line L5 (77.7875, -1.5875) -> (77.7875, -171.45)
  line L6 (-77.7875, -1.5875) -> (-77.7875, -171.45)
  line L7 (-77.7875, -171.45) -> (-77.7875, -1.5875)
  line L8 (0, -171.45) -> (0, -134.620004) construction
  line L9 (77.7875, -171.45) -> (-77.7875, -171.45) construction
  line L10 (77.7875, -171.45) -> (39.6875, -171.45) construction
  line L11 (-77.7875, -171.45) -> (-39.6875, -171.45) construction
  line L12 (39.6875, -171.45) -> (37.30625, -171.45)
  line L13 (37.30625, -171.45) -> (37.30625, -165.1)
  line L14 (37.30625, -165.1) -> (39.6875, -165.1)
  line L15 (39.6875, -165.1) -> (39.6875, -171.45)
  line L16 (33.764904, -171.45) -> (31.383654, -171.45)
  line L17 (31.383654, -171.45) -> (31.383654, -165.1)
  line L18 (31.383654, -165.1) -> (33.764904, -165.1)
  line L19 (33.764904, -165.1) -> (33.764904, -171.45)
  line L20 (27.842308, -171.45) -> (25.461058, -171.45)
  line L21 (25.461058, -171.45) -> (25.461058, -165.1)
  line L22 (25.461058, -165.1) -> (27.842308, -165.1)
  line L23 (27.842308, -165.1) -> (27.842308, -171.45)
  line L24 (21.919712, -171.45) -> (19.538462, -171.45)
  line L25 (19.538462, -171.45) -> (19.538462, -165.1)
  line L26 (19.538462, -165.1) -> (21.919712, -165.1)
  line L27 (21.919712, -165.1) -> (21.919712, -171.45)
  line L28 (15.997115, -171.45) -> (13.615865, -171.45)
  line L29 (13.615865, -171.45) -> (13.615865, -165.1)
  line L30 (13.615865, -165.1) -> (15.997115, -165.1)
  line L31 (15.997115, -165.1) -> (15.997115, -171.45)
  line L32 (10.074519, -171.45) -> (7.693269, -171.45)
  line L33 (7.693269, -171.45) -> (7.693269, -165.1)
  line L34 (7.693269, -165.1) -> (10.074519, -165.1)
  line L35 (10.074519, -165.1) -> (10.074519, -171.45)
  line L36 (4.151923, -171.45) -> (1.770673, -171.45)
  line L37 (1.770673, -171.45) -> (1.770673, -165.1)
  line L38 (1.770673, -165.1) -> (4.151923, -165.1)
  line L39 (4.151923, -165.1) -> (4.151923, -171.45)
  line L40 (-1.770673, -171.45) -> (-4.151923, -171.45)
  line L41 (-4.151923, -171.45) -> (-4.151923, -165.1)
  line L42 (-4.151923, -165.1) -> (-1.770673, -165.1)
  line L43 (-1.770673, -165.1) -> (-1.770673, -171.45)
  line L44 (-7.693269, -171.45) -> (-10.074519, -171.45)
  line L45 (-10.074519, -171.45) -> (-10.074519, -165.1)
  line L46 (-10.074519, -165.1) -> (-7.693269, -165.1)
  line L47 (-7.693269, -165.1) -> (-7.693269, -171.45)
  line L48 (-13.615865, -171.45) -> (-15.997115, -171.45)
  line L49 (-15.997115, -171.45) -> (-15.997115, -165.1)
  line L50 (-15.997115, -165.1) -> (-13.615865, -165.1)
  line L51 (-13.615865, -165.1) -> (-13.615865, -171.45)
  line L52 (-19.538462, -171.45) -> (-21.919712, -171.45)
  line L53 (-21.919712, -171.45) -> (-21.919712, -165.1)
  line L54 (-21.919712, -165.1) -> (-19.538462, -165.1)
  line L55 (-19.538462, -165.1) -> (-19.538462, -171.45)
  line L56 (-25.461058, -171.45) -> (-27.842308, -171.45)
  line L57 (-27.842308, -171.45) -> (-27.842308, -165.1)
  line L58 (-27.842308, -165.1) -> (-25.461058, -165.1)
  line L59 (-25.461058, -165.1) -> (-25.461058, -171.45)
  line L60 (-31.383654, -171.45) -> (-33.764904, -171.45)
  line L61 (-33.764904, -171.45) -> (-33.764904, -165.1)
  line L62 (-33.764904, -165.1) -> (-31.383654, -165.1)
  line L63 (-31.383654, -165.1) -> (-31.383654, -171.45)
  line L64 (-37.30625, -171.45) -> (-39.6875, -171.45)
  line L65 (-39.6875, -171.45) -> (-39.6875, -165.1)
  line L66 (-39.6875, -165.1) -> (-37.30625, -165.1)
  line L67 (-37.30625, -165.1) -> (-37.30625, -171.45)
  dimension "d249" = 38.1
  dimension "d250" = 38.1
  dimension "d251" = 2.38125
  dimension "d252" = 6.35
  dimension "d255" = -76.99375
  dimension "d256" = 0
  constraint midpoint L2 L8.start
  constraint perpendicular L2 L8
  constraint coincident L4.start L5.end
  constraint coincident L6.end L7.start
  constraint perpendicular L4 L10
  constraint perpendicular L6 L11
  constraint horizontal L12
  constraint vertical L13
  constraint horizontal L14
  constraint vertical L15
  measures "d249" distance of L4.start L10.end
  measures "d250" distance of L6.end L11.end
  measures "d252" distance of L10.end L14.end
extrude "Extrude16" cut sketch "Sketch21" against normal up to surface (2.38125 mm away) contours L2 L12 L13 L14 L15 | L2 L64 L65 L66 L67 | L2 L16 L17 L18 L19 | L2 L60 L61 L62 L63 | L2 L20 L21 L22 L23 | L2 L56 L57 L58 L59 | L2 L24 L25 L26 L27 | L2 L52 L53 L54 L55 | L2 L28 L29 L30 L31 | L2 L48 L49 L50 L51 | L2 L32 L33 L34 L35 | L2 L44 L45 L46 L47 | L2 L36 L37 L38 L39 | L2 L40 L41 L42 L43 picked at (38.89375, -169.333333) picked at (-38.89375, -167.216667) picked at (32.971154, -169.333333) picked at (-32.971154, -167.216667) picked at (26.254808, -167.216667) picked at (-27.048558, -167.216667) picked at (20.332212, -167.216667) picked at (-21.125962, -169.333333) picked at (14.409615, -167.216667) picked at (-14.409615, -167.216667) picked at (9.280769, -169.333333) picked at (-9.280769, -167.216667) picked at (3.358173, -169.333333) picked at (-3.358173, -167.216667) bodies 2 in component "enclosure"
ref_plane "WorkPlane1" through (69.05625, 169.06875, 26.19375) normal (0, 1, 0) x (1, 0, 0) in component "rear_panel"
sketch "Sketch1 (3)" plane through (0, 169.06875, 0) normal (0, 1, 0) x (1, 0, 0) in component "rear_panel"
  line L0 (73.2155, -32.54375) -> (39.6875, -32.54375)
  arc A0 (73.2155, -32.54375) -> (75.40625, -30.353) centre (73.2155, -30.353) ccw
  line L1 (75.40625, 30.353) -> (75.40625, -30.353)
  arc A1 (75.40625, 30.353) -> (73.2155, 32.54375) centre (73.2155, 30.353) ccw
  line L2 (-73.2155, 32.54375) -> (73.2155, 32.54375)
  arc A2 (-73.2155, 32.54375) -> (-75.40625, 30.353) centre (-73.2155, 30.353) ccw
  line L3 (-75.40625, -30.353) -> (-75.40625, 30.353)
  arc A3 (-75.40625, -30.353) -> (-73.2155, -32.54375) centre (-73.2155, -30.353) ccw
  line L4 (-39.6875, -32.54375) -> (-73.2155, -32.54375)
  line L5 (-39.6875, -32.54375) -> (39.6875, -32.54375)
extrude "Extrude1'''" add sketch "Sketch1 (3)" along normal blind 2.38125 separate body makes body 9 in component "rear_panel"
sketch "Sketch2 (4)" plane through (0, 171.45, 0) normal (0, 1, 0) x (-1, 0, 0) in component "rear_panel"
  arc A0 (75.40625, 30.353) -> (73.2155, 32.54375) centre (73.2155, 30.353) ccw
  line L0 (73.2155, 32.54375) -> (-73.2155, 32.54375)
  arc A1 (-73.2155, 32.54375) -> (-75.40625, 30.353) centre (-73.2155, 30.353) ccw
  line L1 (-75.40625, 30.353) -> (-75.40625, -30.353)
  arc A2 (-75.40625, -30.353) -> (-73.2155, -32.54375) centre (-73.2155, -30.353) ccw
  line L2 (-73.2155, -32.54375) -> (73.2155, -32.54375)
  arc A3 (73.2155, -32.54375) -> (75.40625, -30.353) centre (73.2155, -30.353) ccw
  line L3 (75.40625, -30.353) -> (75.40625, 30.353)
  line L4 (-39.6875, 32.54375) -> (-39.6875, 34.925)
  line L5 (-39.6875, 34.925) -> (-39.6875, 32.54375)
  line L6 (-39.6875, 32.54375) -> (-37.30625, 32.54375)
  line L7 (-37.30625, 32.54375) -> (-37.30625, 28.575)
  line L8 (-37.30625, 28.575) -> (-39.6875, 28.575)
  line L9 (-39.6875, 28.575) -> (-39.6875, 32.54375)
  line L10 (-33.764904, 32.54375) -> (-31.383654, 32.54375)
  line L11 (-33.764904, 28.575) -> (-33.764904, 32.54375)
  line L12 (-31.383654, 32.54375) -> (-31.383654, 28.575)
  line L13 (-31.383654, 28.575) -> (-33.764904, 28.575)
  line L14 (-27.842308, 32.54375) -> (-25.461058, 32.54375)
  line L15 (-27.842308, 28.575) -> (-27.842308, 32.54375)
  line L16 (-25.461058, 32.54375) -> (-25.461058, 28.575)
  line L17 (-25.461058, 28.575) -> (-27.842308, 28.575)
  line L18 (-21.919712, 32.54375) -> (-19.538462, 32.54375)
  line L19 (-21.919712, 28.575) -> (-21.919712, 32.54375)
  line L20 (-19.538462, 32.54375) -> (-19.538462, 28.575)
  line L21 (-19.538462, 28.575) -> (-21.919712, 28.575)
  line L22 (-15.997115, 32.54375) -> (-13.615865, 32.54375)
  line L23 (-15.997115, 28.575) -> (-15.997115, 32.54375)
  line L24 (-13.615865, 32.54375) -> (-13.615865, 28.575)
  line L25 (-13.615865, 28.575) -> (-15.997115, 28.575)
  line L26 (-10.074519, 32.54375) -> (-7.693269, 32.54375)
  line L27 (-10.074519, 28.575) -> (-10.074519, 32.54375)
  line L28 (-7.693269, 32.54375) -> (-7.693269, 28.575)
  line L29 (-7.693269, 28.575) -> (-10.074519, 28.575)
  line L30 (-4.151923, 32.54375) -> (-1.770673, 32.54375)
  line L31 (-4.151923, 28.575) -> (-4.151923, 32.54375)
  line L32 (-1.770673, 32.54375) -> (-1.770673, 28.575)
  line L33 (-1.770673, 28.575) -> (-4.151923, 28.575)
  line L34 (1.770673, 32.54375) -> (4.151923, 32.54375)
  line L35 (1.770673, 28.575) -> (1.770673, 32.54375)
  line L36 (4.151923, 32.54375) -> (4.151923, 28.575)
  line L37 (4.151923, 28.575) -> (1.770673, 28.575)
  line L38 (7.693269, 32.54375) -> (10.074519, 32.54375)
  line L39 (7.693269, 28.575) -> (7.693269, 32.54375)
  line L40 (10.074519, 32.54375) -> (10.074519, 28.575)
  line L41 (10.074519, 28.575) -> (7.693269, 28.575)
  line L42 (13.615865, 32.54375) -> (15.997115, 32.54375)
  line L43 (13.615865, 28.575) -> (13.615865, 32.54375)
  line L44 (15.997115, 32.54375) -> (15.997115, 28.575)
  line L45 (15.997115, 28.575) -> (13.615865, 28.575)
  line L46 (19.538462, 32.54375) -> (21.919712, 32.54375)
  line L47 (19.538462, 28.575) -> (19.538462, 32.54375)
  line L48 (21.919712, 32.54375) -> (21.919712, 28.575)
  line L49 (21.919712, 28.575) -> (19.538462, 28.575)
  line L50 (25.461058, 32.54375) -> (27.842308, 32.54375)
  line L51 (25.461058, 28.575) -> (25.461058, 32.54375)
  line L52 (27.842308, 32.54375) -> (27.842308, 28.575)
  line L53 (27.842308, 28.575) -> (25.461058, 28.575)
  line L54 (31.383654, 32.54375) -> (33.764904, 32.54375)
  line L55 (31.383654, 28.575) -> (31.383654, 32.54375)
  line L56 (33.764904, 32.54375) -> (33.764904, 28.575)
  line L57 (33.764904, 28.575) -> (31.383654, 28.575)
  line L58 (37.30625, 32.54375) -> (39.6875, 32.54375)
  line L59 (37.30625, 28.575) -> (37.30625, 32.54375)
  line L60 (39.6875, 32.54375) -> (39.6875, 28.575)
  line L61 (39.6875, 28.575) -> (37.30625, 28.575)
  dimension "d262" = 2.38125
  dimension "d263" = 3.96875
  dimension "d266" = 76.99375
  dimension "d267" = 0
  constraint horizontal L6
  constraint vertical L7
  constraint horizontal L8
  constraint vertical L9